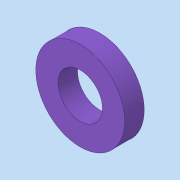
# Autodesk Inventor part: ArduinoSpacers
Saved by Autodesk Inventor 2017 (Build 210142000, 142)
## iProperties
Created: 2017-04-22
Part Number: ArduinoSpacers
Material: ABS Plastic
Document SubType Name: Modeling
Designer: Derek Wider
Mass: 0.0607522 g
Surface Area: 1.1971 cm^2
Volume: 0.0573134 cm^3
Density: 1.06 g/cm^3
Appearance: Violet
Author: Derek Wider
Autodesk Inventor part; units mm, degrees
ref_plane "YZ Plane" through (0, 0, 0) normal (1, 0, 0) x (0, 1, 0)
ref_plane "XZ Plane" through (0, 0, 0) normal (0, 1, 0) x (-1, 0, 0)
ref_plane "XY Plane" through (0, 0, 0) normal (0, 0, 1) x (1, 0, 0)
sketch "Sketch1" plane through (0, 0, 0) normal (0, 0, 1) x (1, 0, 0)
  circle A0 centre (0, 0) radius 1.5875
  circle A1 centre (0, 0) radius 3.175
  dimension "d0" = 3.175
  dimension "d1" = 6.35
  constraints: 2 centre point, 2 coincident
  measures "d0" diameter of A0
  measures "d1" diameter of A1
extrude "Extrusion1" add sketch "Sketch1" along normal blind 1.397
body "Solid1"
